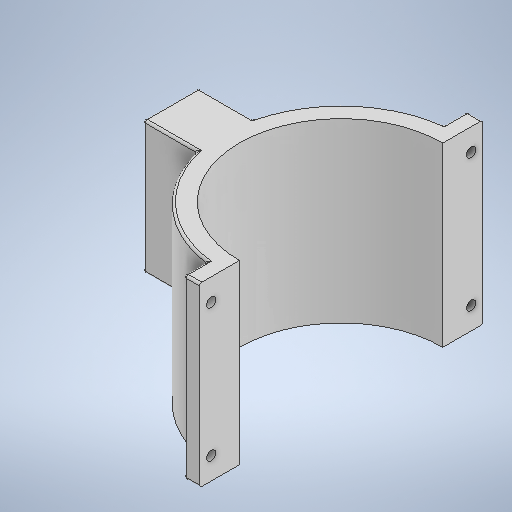
# Autodesk Inventor part: moror-mount1
Saved by Autodesk Inventor 2025.2 (Build 292293000, 293)
## iProperties
Created: 2025-02-07
Part Number: moror-mount1
Material: 一般
Document SubType Name: Modeling
Designer: mahhy
Density: 1 g/cm^3
Appearance: 既定
Author: mahhy
## iProperties of the stored document moror-mount1_3D プリント.ipt
Created: 2025-02-16
Part Number: moror-mount1_3D プリント
Material: 一般
Document SubType Name: Modeling
Designer: mahhy
Density: 1 g/cm^3
Appearance: 既定
Author: mahhy
Autodesk Inventor part; units mm, degrees
ref_plane "YZ Plane" through (0, 0, 0) normal (1, 0, 0) x (0, 1, 0)
ref_plane "XZ Plane" through (0, 0, 0) normal (0, 1, 0) x (-1, 0, 0)
ref_plane "XY Plane" through (0, 0, 0) normal (0, 0, 1) x (1, 0, 0)
sketch "スケッチ1" plane through (0, 0, 0) normal (0, 1, 0) x (-1, 0, 0)
  line L0 (0, 0) -> (60, 0)
  line L1 (60, 0) -> (60, -120)
  line L2 (60, -120) -> (0, -120)
  line L3 (0, -120) -> (0, 0)
  circle A0 centre (0, -60) radius 46
  circle A1 centre (0, -60) radius 54
  line L4 (0, -14) -> (7, -14)
  line L5 (7, -14) -> (7, 4)
  line L6 (7, 4) -> (0, 4)
  line L7 (0, 4) -> (0, -14)
  line L8 (0, -106) -> (7, -106)
  line L9 (7, -106) -> (7, -124)
  line L10 (7, -124) -> (0, -124)
  line L11 (0, -124) -> (0, -106)
  line L12 (54, -47.5) -> (46, -47.5)
  line L13 (46, -47.5) -> (46, -72.5)
  line L14 (46, -72.5) -> (54, -72.5)
  line L15 (54, -72.5) -> (54, -47.5)
  point P0 (46, -60)
  point P1 (52.5333, -47.5)
  point P2 (7, -6.4556)
  point P3 (0, -2)
  point P4 (0, -118)
  point P5 (7, -113.5444)
  point P6 (52.5333, -72.5)
  point P7 (7, 0)
  point P8 (7, -120)
  point P9 (54, -60)
  point P10 (0, -114)
  point P11 (0, -6)
  point P12 (54, -60)
  dimension "d2" = 60
  dimension "d3" = 120
  dimension "d4" = 92
  dimension "d5" = 108
  dimension "d6" = 7
  dimension "d7" = 18
  dimension "d8" = 7
  dimension "d9" = 18
  dimension "d10" = 8
  dimension "d11" = 25
  constraints: 32 end point, 8 parallel, 4 horizontal, 4 perpendicular, 3 midpoint, 3 point on circle, 2 centre point, 2 point on line, 1 coincident, 1 horizontal alignment
  measures "d2" distance of L1.end L2.end
  measures "d3" distance of L0.end L1.end
  measures "d4" diameter of A0
  measures "d5" diameter of A1
  measures "d6" distance of L6.end L5.end
  measures "d7" distance of L5.end L4.end
  measures "d8" distance of L9.end L10.end
  measures "d9" distance of L8.end L9.end
  measures "d10" distance of L14.end L13.end
  measures "d11" distance of L13.end L12.end
extrude "押し出し1" add sketch "スケッチ1" along normal blind 80 contours L7 L6 L5 L0 | L0 L5 A1 L3 | A1 L5 L4 L3 | A1 L12 L13 A0 L4 L5 | A1 L9 L2 L3 | L3 L8 L9 A1 | L12 L15 A1 | A1 L14 L13 L12 | A0 L13 L14 A1 L9 L8 | L2 L9 L10 L11 | L15 L14 A1
sketch "スケッチ2" plane through (-54, 0, -72.5) normal (-1, 0, 0) x (0, 0, 1)
  line L0 (25, 0) -> (25, 80) projected
  line L1 (0, 20) -> (25, 20)
  line L2 (25, 20) -> (25, 80)
  line L3 (25, 80) -> (0, 80)
  line L4 (0, 80) -> (0, 20)
  line L5 (0, 0) -> (25, 0) projected
  line L6 (-33.5, 80) -> (58.5, 80) projected
  point P0 (72.5, 0)
  point P1 (25, 20)
  point P2 (12.5, 0)
  point P3 (12.5, 80)
  dimension "d14" = 25
  dimension "d15" = 60
  constraints: 8 end point, 2 parallel, 1 horizontal, 1 midpoint, 1 perpendicular
  measures "d14" distance of L3.end L0.end
  measures "d15" distance of L0.end L1.end
extrude "押し出し2" add sketch "スケッチ2" along normal blind 23
sketch "スケッチ3" plane through (-77, 0, -72.5) normal (-1, 0, 0) x (0, 0, 1)
  line L0 (7.65, 75) -> (17.35, 75)
  line L1 (7.65, 26.1) -> (17.35, 26.1)
  line L2 (25, 80) -> (0, 80) projected
  line L3 (0, 20) -> (25, 20) projected
  point P0 (72.5, 0)
  point P1 (12.5, 26.1)
  point P2 (12.5, 30.1)
  point P3 (12.5, 80)
  point P4 (12.5, 75)
  point P5 (12.5, 80)
  dimension "d23" = 9.7
  dimension "d24" = 9.7
  dimension "d30" = 0
  dimension "d101" = 5
  dimension "d102" = 6.1
  constraints: 4 end point, 4 midpoint, 1 parallel, 1 vertical alignment
  measures "d23" distance of L0.end L0.start
  measures "d24" distance of L1.end L1.start
  measures "d30" horizontal distance of point (12.5, 30.1) point (12.5, 26.1)
  measures "d101" distance between parallel lines of L2 L0
  measures "d102" distance between parallel lines of L3 L1
hole "穴1" at (-77, 75, -64.85) at (-77, 75, -55.15) at (-77, 26.1, -55.15) at (-77, 26.1, -64.85) direction (1, 0, 0) diameter 4 depth 5
sketch "スケッチ5" plane through (-7, 0, -124) normal (-1, 0, 0) x (0, 0, 1)
  line L0 (0, 80) -> (10.4556, 80) projected
  line L1 (18, 0) -> (0, 0) projected
  line L2 (128, 80) -> (110, 80) projected
  line L3 (117.5444, 0) -> (128, 0) projected
  line L4 (117.5444, 80) -> (128, 80) projected
  line L5 (0, 0) -> (10.4556, 0) projected
  point P0 (5.2278, 80)
  point P1 (5.2278, 70)
  point P2 (122.7722, 70)
  point P3 (122.7722, 10)
  point P4 (5.2278, 80)
  point P5 (122.7722, 0)
  point P6 (122.7722, 80)
  point P7 (5.2278, 80)
  point P8 (122.7722, 80)
  point P9 (122.7722, 0)
  point P10 (5.2278, 10)
  point P11 (5.2278, 0)
  dimension "d56" = 10
  dimension "d58" = 10
  dimension "d59" = 10
  dimension "d67" = 0
  dimension "d68" = 0
  dimension "d69" = 0
  dimension "d70" = 10
  constraints: 8 midpoint
  measures "d56" distance of point (5.228, 80) point (5.228, 70)
  measures "d58" distance of point (122.772, 0) point (122.772, 10)
  measures "d59" distance of point (122.772, 70) point (122.772, 80)
  measures "d67" horizontal distance of point (5.228, 70) point (5.228, 80)
  measures "d68" horizontal distance of point (122.772, 70) point (122.772, 80)
  measures "d69" horizontal distance of point (122.772, 0) point (122.772, 10)
  measures "d70" distance of point (5.228, 0) point (5.228, 10)
hole "穴3" at (-7, 70, -118.7722) at (-7, 10, -1.2278) at (-7, 70, -1.2278) at (-7, 10, -118.7722) direction (1, 0, 0) diameter 4.2 end through all
fillet "フィレット1" radius 1 14 edges at (-3.5, 80, -124) (-7, 80, -118.7722) (-7, 40, -124) (-7, 0, -118.7722) (-3.5, 0, -124) (-36.1554, 80, -100.1097) (-36.1554, 0, -100.1097) (-36.1554, 80, -19.8903) (-7, 80, -1.2278) (-3.5, 80, 4) (-7, 40, 4) (-36.1554, 0, -19.8903) (-7, 0, -1.2278) (-3.5, 0, 4)
fillet "フィレット2" radius 2 1 edges at (-54, 0, -60)
fillet "フィレット4" radius 1 10 edges at (-77, 50, -47.5) (-77, 80, -60) (-77, 50, -72.5) (-77, 20, -60) (-65.5, 20, -47.5) (-52.0191, 80, -47.5) (-64.7667, 80, -47.5) (-65.5, 20, -72.5) (-52.0191, 80, -72.5) (-64.7667, 80, -72.5)
fillet "フィレット5" radius 1 12 edges at (-52.2762, 79.7376, -72.1753) (-52.2296, 0.2903, -72.5) (-52.5333, 40, -72.5) (-6.669, 79.7433, -113.253) (-6.669, 0.2567, -113.253) (-7, 40, -113.5444) (-52.2762, 79.7375, -47.8247) (-52.2296, 0.2903, -47.5) (-52.5333, 40, -47.5) (-6.669, 79.7433, -6.747) (-6.669, 0.2567, -6.747) (-7, 40, -6.4556)
sketch "スケッチ9" plane through (-77, 0, -72.5) normal (-1, 0, 0) x (0, 0, 1)
  line L0 (2.45, 70.2) -> (22.55, 70.2)
  line L1 (22.55, 70.2) -> (22.55, 30.1)
  line L2 (22.55, 30.1) -> (2.45, 30.1)
  line L3 (2.45, 30.1) -> (2.45, 70.2)
  line L4 (1, 79) -> (24, 79) projected
  line L5 (24, 80) -> (1, 80) projected
  line L6 (-50.5, 1) -> (-50.5, 79) projected
  point P0 (72.5, 0)
  point P1 (12.5, 70.2)
  point P2 (12.5, 79)
  point P3 (12.5, 40)
  point P4 (12.5, 30.1)
  point P5 (-50.5, 40)
  dimension "d103" = 20.1
  dimension "d104" = 40.1
  dimension "d106" = 9.9
  constraints: 8 end point, 4 midpoint, 2 parallel, 2 vertical alignment, 1 horizontal, 1 horizontal alignment, 1 perpendicular
  measures "d103" distance of L1.end L2.end
  measures "d104" distance of L0.end L1.end
  measures "d106" distance from line of L2 point (12.5, 40)
extrude "押し出し6" cut sketch "スケッチ9" against normal blind 28
